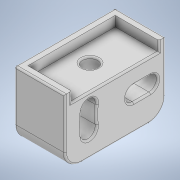
# Autodesk Inventor part: hoop_mount
Saved by Autodesk Inventor 2022 (Build 260153000, 153)
## iProperties
Created: 2022-03-04
Part Number: hoop_mount
Material: Generic
Document SubType Name: Modeling
Designer: Frey
Density: 1 g/cm^3
Appearance: Default
Author: Frey
Autodesk Inventor part; units mm, degrees
ref_plane "YZ Plane" through (0, 0, 0) normal (1, 0, 0) x (0, 1, 0)
ref_plane "XZ Plane" through (0, 0, 0) normal (0, 1, 0) x (-1, 0, 0)
ref_plane "XY Plane" through (0, 0, 0) normal (0, 0, 1) x (1, 0, 0)
sketch "Sketch1" plane through (0, 0, 0) normal (1, 0, 0) x (0, 1, 0)
  line L0 (10, 15) -> (-10, 15)
  line L1 (-10, 15) -> (-10, -15)
  line L2 (-10, -15) -> (10, -15)
  line L3 (10, -15) -> (10, 15)
  line L4 (10, 15) -> (-10, -15) construction
  line L5 (10, -15) -> (-10, 15) construction
  point P0 (0, 0)
  point P1 (0, 0)
  dimension "d0" = 20
  dimension "d1" = 30
  constraints: 12 end point, 2 parallel, 1 coincident, 1 horizontal, 1 midpoint, 1 perpendicular
  measures "d0" distance of L1.end L2.end
  measures "d1" distance between parallel lines of L0 L2
extrude "Extrusion1" add sketch "Sketch1" along normal blind 15
sketch "Sketch2" plane through (0, 10, 15) normal (0, 1, 0) x (1, 0, 0)
  line L0 (15, 30) -> (15, 0) projected
  line L1 (2, 2) -> (2, 28)
  line L2 (2, 2) -> (15, 2)
  line L3 (2, 28) -> (15, 28)
  line L4 (15, 0) -> (15, 30) projected
  line L5 (0, 0) -> (15, 0) projected
  line L6 (0, 30) -> (15, 30) projected
  point P0 (0, 15)
  dimension "d4" = 2
  dimension "d5" = 2
  dimension "d6" = 2
  constraints: 6 end point, 2 point on line, 1 horizontal, 1 perpendicular, 1 vertical alignment
  measures "d4" distance from line of L1 point (0, 15)
  measures "d5" distance between parallel lines of L5 L2
  measures "d6" distance between parallel lines of L6 L3
extrude "Extrusion2" cut sketch "Sketch2" against normal blind 3
sketch "Sketch3" plane through (0, -10, -15) normal (0, -1, 0) x (1, 0, 0)
  line L0 (11, 12.9793) -> (7.5, 10.9585)
  line L1 (7.5, 10.9585) -> (4, 12.9793)
  line L2 (4, 12.9793) -> (4, 17.0207)
  line L3 (4, 17.0207) -> (7.5, 19.0415)
  line L4 (7.5, 19.0415) -> (11, 17.0207)
  line L5 (11, 17.0207) -> (11, 12.9793)
  line L6 (0, 30) -> (0, 0) projected
  line L7 (15, 30) -> (15, 0) projected
  point P0 (0, 15)
  point P1 (7.5, 15)
  point P2 (0, 15)
  dimension "d9" = 15
  dimension "d10" = 7.5
  dimension "d11" = 7
  constraints: 12 end point, 2 horizontal alignment, 1 midpoint, 1 vertical alignment, 13 other
  measures "d9" distance between parallel lines of L6 L7
  measures "d10" distance of point (0, 15) point (7.5, 15)
  measures "d11" distance between parallel lines of L2 L5
extrude "Extrusion3" cut sketch "Sketch3" against normal blind 5
sketch "Sketch4" plane through (0, -5, -15) normal (0, -1, 0) x (1, 0, 0)
  circle A0 centre (7.5, 15) radius 2.25
  line L0 (15, 2) -> (15, 28) projected
  point P0 (0, 15)
  dimension "d14" = 7.5
  dimension "d15" = 4.5
  constraints: 1 centre point
  measures "d14" distance from line of A0.centre L0
  measures "d15" diameter of A0
extrude "Extrusion4" cut sketch "Sketch4" against normal up to surface (12 mm away)
sketch "Sketch5" plane through (15, 0, 0) normal (1, 0, 0) x (0, 0, -1)
  line L0 (5.5, 0) -> (10.5, 0) construction
  line L1 (5.5, 2.25) -> (10.5, 2.25)
  line L2 (10.5, -2.25) -> (5.5, -2.25)
  arc A0 (5.5, 2.25) -> (5.5, -2.25) centre (5.5, 0) ccw
  arc A1 (10.5, -2.25) -> (10.5, 2.25) centre (10.5, 0) ccw
  arc A2 (-7.7162, 3) -> (-7.7162, -3) centre (8, 0) ccw construction
  arc A3 (-9.9263, 3.4219) -> (-9.9263, -3.4219) centre (8, 0) ccw
  arc A4 (-5.5061, 2.5781) -> (-5.5061, -2.5781) centre (8, 0) ccw
  arc A5 (-5.5061, 2.5781) -> (-9.9263, 3.4219) centre (-7.7162, 3) ccw
  arc A6 (-9.9263, -3.4219) -> (-5.5061, -2.5781) centre (-7.7162, -3) ccw
  point P0 (0, 0)
  point P1 (8, 0)
  point P2 (-8, 0)
  dimension "d18" = 4.5
  dimension "d25" = 4.5
  dimension "d26" = 6
  dimension "d27" = 16
  dimension "d28" = 16
  dimension "d29" = 8
  dimension "d30" = 5
  constraints: 15 point on circle, 8 end point, 8 tangent, 7 centre point, 2 coincident, 2 horizontal alignment, 1 horizontal, 1 midpoint, 1 parallel, 1 vertical alignment
  measures "d18" distance between parallel lines of L2 L1
  measures "d25" radial gap between concentric circles of A4 A3
  measures "d26" distance of point (-7.716, -3) point (-7.716, 3)
  measures "d27" radius of A2
  measures "d28" distance of point (8, 0) point (-8, 0)
  measures "d29" distance of point (-8, 0) point (0, 0)
  measures "d30" distance of L0.end L0.start
extrude "Extrusion5" cut sketch "Sketch5" against normal up to surface (15 mm away)
fillet "Fillet1" radius 5 2 edges at (7.5, -10, 15) (7.5, -10, -15)
fillet "Fillet2" radius 0.5 40 edges at (0, -8.5355, 13.5355) (0, -10, 0) (0, -8.5355, -13.5355) (0, 2.5, -15) (0, 2.5, 15) (0, -5.2101, 7.2944) (0, 0, 5.75) (0, 5.2101, 7.2944) (0, 0, 10.25) (0, -2.25, -8) (0, 0, -12.75) (0, 2.25, -8) (0, 0, -3.25) (7.5, 10, 15) (0, 10, 0) (7.5, 10, -15) (15, -5.2101, 7.2944) (15, 0, 10.25) (15, 5.2101, 7.2944) (15, 0, 5.75) (15, 2.25, -8) (15, 0, -12.75) (15, -2.25, -8) (15, 0, -3.25) (15, -8.5355, 13.5355) (15, -10, 0) (15, -8.5355, -13.5355) (15, 2.5, -15) (15, 2.5, 15) (15, 7, 0) (15, 8.5, -13) (15, 8.5, 13) (5.25, 7, 0) (5.25, -5, 0) (5.75, -10, -3.0311) (9.25, -10, -3.0311) (11, -10, 0) (9.25, -10, 3.0311) (5.75, -10, 3.0311) (4, -10, 0)
body "Solid1"
